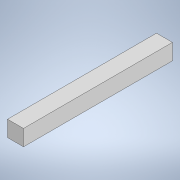
# Autodesk Inventor part: legs
Saved by Autodesk Inventor 2020.2 (Build 242310000, 310)
## iProperties
Created: 2020-04-15
Part Number: legs
Material: Generic
Document SubType Name: Modeling
Designer: tanma
Density: 1 g/cm^3
Appearance: Default
Author: tanma
Autodesk Inventor part; units mm, degrees
ref_plane "YZ Plane" through (0, 0, 0) normal (1, 0, 0) x (0, 1, 0)
ref_plane "XZ Plane" through (0, 0, 0) normal (0, 1, 0) x (-1, 0, 0)
ref_plane "XY Plane" through (0, 0, 0) normal (0, 0, 1) x (1, 0, 0)
sketch "Sketch3" plane through (0, 0, 0) normal (0, 0, 1) x (1, 0, 0)
  line L0 (-0.375, -0.375) -> (0.375, -0.375)
  line L1 (0.375, -0.375) -> (0.375, 0.375)
  line L2 (0.375, 0.375) -> (-0.375, 0.375)
  line L3 (-0.375, 0.375) -> (-0.375, -0.375)
  line L4 (-0.375, -0.375) -> (0.375, 0.375) construction
  line L5 (0.375, -0.375) -> (-0.375, 0.375) construction
  point P0 (0, 0)
  dimension "d10" = 0.75
  dimension "d11" = 0.75
  constraints: 12 end point, 2 midpoint, 2 parallel, 1 horizontal, 1 perpendicular
  measures "d10" distance of L1.end L2.end
  measures "d11" distance of L0.end L1.end
extrude "Extrusion3" add sketch "Sketch3" against normal blind 7
body "Solid2"
